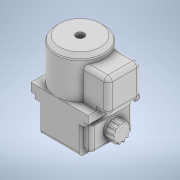
# Autodesk Inventor part: EG_Vacuumpump
Saved by Autodesk Inventor 2022 (Build 260153000, 153)
## iProperties
Created: 2023-07-06
Part Number: EG_Vacuumpump
Material: Generic
Document SubType Name: Modeling
Designer: grees
Density: 1 g/cm^3
Appearance: Default
Author: grees
Autodesk Inventor part; units mm, degrees
ref_plane "YZ Plane" through (0, 0, 0) normal (1, 0, 0) x (0, 1, 0)
ref_plane "XZ Plane" through (0, 0, 0) normal (0, 1, 0) x (-1, 0, 0)
ref_plane "XY Plane" through (0, 0, 0) normal (0, 0, 1) x (1, 0, 0)
sketch "Sketch1" plane through (0, 0, 0) normal (0, 1, 0) x (-1, 0, 0)
  circle A0 centre (0, 0) radius 30
  dimension "d0" = 60
  constraints: 1 centre point, 1 coincident
  measures "d0" diameter of A0
extrude "Extrusion1" add sketch "Sketch1" along normal blind 10
chamfer "Chamfer1" distance 5 angle 45 1 edges at (30, 10, 0)
sketch "Sketch2" plane through (0, 0, 0) normal (0, -1, 0) x (1, 0, 0)
  circle A0 centre (0, 0) radius 30
  dimension "d9" = 60
  constraints: 1 centre point, 1 coincident
  measures "d9" diameter of A0
extrude "Extrusion2" add sketch "Sketch2" along normal blind 40
chamfer "Chamfer3" distance 1 angle 45 1 edges at (30, 5, 0)
sketch "Sketch3" plane through (0, -40, 0) normal (0, -1, 0) x (1, 0, 0)
  circle A0 centre (0, 0) radius 30 projected
  line L0 (-30, 0) -> (-30, 30)
  line L1 (-30, 0) -> (-30, -30)
  line L2 (-30, -30) -> (40, -30)
  line L3 (40, -30) -> (40, 30)
  line L4 (40, 30) -> (-30, 30)
  dimension "d15" = 30
  dimension "d16" = 30
  dimension "d17" = 70
  dimension "d18" = 60
  constraints: 10 end point, 3 vertical, 2 perpendicular, 1 horizontal alignment, 1 other
  measures "d15" distance of L0.start L0.end
  measures "d16" distance of L0.start L1.end
  measures "d17" distance of L1.end L2.end
  measures "d18" distance of L2.end L3.end
extrude "Extrusion3" add sketch "Sketch3" along normal blind 10
sketch "Sketch4" plane through (0, -50, 0) normal (0, -1, 0) x (1, 0, 0)
  line L0 (40, 30) -> (-30, 30) projected
  line L1 (-30, 30) -> (-25, 30)
  line L2 (-25, 30) -> (-25, -30)
  line L3 (-30, -30) -> (40, -30) projected
  line L4 (-25, -30) -> (35, -30)
  line L5 (0, -30) -> (40, -30) projected
  line L6 (35, -30) -> (35, 30)
  line L7 (35, 30) -> (-25, 30)
  point P0 (0, 0)
  dimension "d21" = 5
  dimension "d22" = 60
  constraints: 10 end point, 4 point on line, 2 perpendicular, 1 collinear
  measures "d21" distance of L0.end L1.end
  measures "d22" distance of L2.end L4.end
extrude "Extrusion4" add sketch "Sketch4" along normal blind 5
sketch "Sketch5" plane through (0, -55, 0) normal (0, -1, 0) x (1, 0, 0)
  line L0 (-25, -30) -> (-25, 30) projected
  line L1 (-25, 30) -> (-18, 30)
  line L2 (0, 30) -> (-30, 30) projected
  line L3 (-18, 30) -> (-18, -30)
  line L4 (-25, -30) -> (35, -30) projected
  line L5 (-18, -30) -> (29, -30)
  line L6 (29, -30) -> (29, 30)
  line L7 (40, 30) -> (0, 30) projected
  line L8 (29, 30) -> (-18, 30)
  point P0 (0, 0)
  dimension "d25" = 7
  dimension "d26" = 47
  constraints: 10 end point, 4 point on line, 3 perpendicular
  measures "d25" distance of L0.end L1.end
  measures "d26" distance of L3.end L5.end
extrude "Extrusion5" add sketch "Sketch5" along normal blind 35 contours L3 L2 L7 L6 L4
fillet "Fillet1" radius 5 1 edges at (5.5, -90, 30)
fillet "Fillet2" radius 5 1 edges at (5.5, -90, -30)
sketch "Sketch6" plane through (0, -90, 0) normal (0, -1, 0) x (1, 0, 0)
  circle A0 centre (0, 0) radius 10
  dimension "d31" = 20
  constraints: 1 centre point, 1 coincident
  measures "d31" diameter of A0
extrude "Extrusion6" cut sketch "Sketch6" against normal blind 35
sketch "Sketch7" plane through (29, -55, 30) normal (1, 0, 0) x (0, 0, -1)
  line L0 (0, 0) -> (0, -35) projected
  line L1 (0, 0) -> (5, 0)
  line L2 (40, 0) -> (20, 0) projected
  line L3 (5, 0) -> (5, -30)
  line L4 (5, -30) -> (55, -30)
  line L5 (55, -30) -> (55, 0)
  line L6 (0, 0) -> (60, 0) projected
  line L7 (55, 0) -> (5, 0)
  point P0 (30, 55)
  point P1 (0, -30)
  dimension "d34" = 5
  constraints: 10 end point, 3 perpendicular, 1 collinear, 1 point on line
  measures "d34" distance of L0.start L1.end
extrude "Extrusion7" add sketch "Sketch7" along normal blind 10
fillet "Fillet3" radius 4 1 edges at (39, -70, 25)
fillet "Fillet4" radius 4 3 edges at (39, -85, -2) (37.8284, -85, 23.8284) (32, -85, 25)
fillet "Fillet5" radius 4 3 edges at (39, -68, -25) (37.8284, -83.8284, -25) (32, -85, -25)
sketch "Sketch8" plane through (39, -55, 30) normal (1, 0, 0) x (0, 0, -1)
  circle A0 centre (30, -12.943) radius 10
  point P0 (30, 55)
  dimension "d40" = 20
  constraints: 1 centre point
  measures "d40" diameter of A0
extrude "Extrusion8" cut sketch "Sketch8" against normal blind 45
sketch "Sketch9" plane through (39, -55, 30) normal (1, 0, 0) x (0, 0, -1)
  circle A0 centre (30, -13.3001) radius 7.5
  point P0 (30, 55)
  dimension "d43" = 15
  constraints: 1 centre point
  measures "d43" diameter of A0
extrude "Extrusion10" add sketch "Sketch9" against normal blind 50
sketch "Sketch10" plane through (39, -55, 30) normal (1, 0, 0) x (0, 0, -1)
  circle A0 centre (30, -12.943) radius 11
  point P0 (30, 55)
  dimension "d48" = 22
  constraints: 1 centre point
  measures "d48" diameter of A0
extrude "Extrusion11" add sketch "Sketch10" along normal blind 2
sketch "Sketch11" plane through (41, -67.943, 0) normal (1, 0, 0) x (0, 0, -1)
  circle A0 centre (0, -0.3571) radius 7.5 projected
  circle A1 centre (0, -0.3571) radius 11
  point P0 (0, 67.943)
  dimension "d51" = 22
  constraints: 1 centre point, 1 coincident
  measures "d51" diameter of A1
extrude "Extrusion12" add sketch "Sketch11" along normal blind 10 contours A0 | A1
sketch "Sketch12" plane through (51, -68.3001, 0) normal (1, 0, 0) x (0, 0, -1)
  circle A0 centre (0, 0.3571) radius 11 projected
  line L0 (0, 11.3571) -> (0, -10.6429)
  circle A1 centre (0, 11.3571) radius 2
  circle A2 centre (-5.5, 9.8834) radius 2
  circle A3 centre (-9.5263, 5.8571) radius 2
  circle A4 centre (-11, 0.3571) radius 2
  circle A5 centre (-9.5263, -5.1429) radius 2
  circle A6 centre (-5.5, -9.1692) radius 2
  circle A7 centre (0, -10.6429) radius 2
  circle A8 centre (5.5, -9.1692) radius 2
  circle A9 centre (9.5263, -5.1429) radius 2
  circle A10 centre (11, 0.3571) radius 2
  circle A11 centre (9.5263, 5.8571) radius 2
  circle A12 centre (5.5, 9.8834) radius 2
  point P0 (0, 68.3001)
  dimension "d57" = 360
  constraints: 12 centre point, 2 end point, 2 point on circle, 1 coincident, 1 vertical, 25 other
extrude "Extrusion13" cut sketch "Sketch12" against normal blind 10 contours A0 A10 | A0 A10 | A11 A0 | A0 A11 | A9 A0 | A0 A9 | A12 A0 | A0 A12 | A8 A0 | A0 A8 | A1 L0 A0 | A0 A1 | A7 A0 | A0 L0 A7 | L0 A1 A0 | A0 A7 L0 | A2 A0 | A0 A2 | A6 A0 | A0 A6 | A3 A0 | A0 A3 | A5 A0 | A0 A5 | A4 A0 | A0 A4
sketch "Sketch13" plane through (0, -90, 0) normal (0, -1, 0) x (1, 0, 0)
  circle A0 centre (0, 0) radius 11.5
  dimension "d61" = 23
  constraints: 1 centre point, 1 coincident
  measures "d61" diameter of A0
extrude "Extrusion14" add sketch "Sketch13" along normal blind 4
sketch "Sketch14" plane through (0, -94, 0) normal (0, -1, 0) x (1, 0, 0)
  circle A0 centre (0, 0) radius 10
  dimension "d64" = 20
  constraints: 1 centre point, 1 coincident
  measures "d64" diameter of A0
extrude "Extrusion15" cut sketch "Sketch14" against normal blind 5
sketch "Sketch15" plane through (40, -40, 30) normal (1, 0, 0) x (0, 0, -1)
  circle A0 centre (54.5126, -5.7503) radius 2.5
  point P0 (30, 40)
  dimension "d67" = 5
  constraints: 1 centre point
  measures "d67" diameter of A0
extrude "Extrusion16" add sketch "Sketch15" along normal blind 2
sketch "Sketch16" plane through (40, -40, 30) normal (1, 0, 0) x (0, 0, -1)
  circle A0 centre (54.5126, -5.7503) radius 2.5 projected
  circle A1 centre (54.5126, -5.7503) radius 4
  point P0 (30, 40)
  dimension "d70" = 8
  constraints: 1 centre point, 1 coincident
  measures "d70" diameter of A1
extrude "Extrusion18" add sketch "Sketch16" along normal blind 6 contours A0 | A1
fillet "Fillet6" radius 1.5 1 edges at (46, -45.7503, -20.5126)
sketch "Sketch18" plane through (0, -40, 0) normal (0, 1, 0) x (1, 0, 0)
  line L0 (24.2354, 0) -> (24.2354, 20)
  line L1 (24.2354, 0) -> (44.2354, 0) construction
  line L2 (24.2354, 0) -> (24.2354, -20)
  line L3 (40, -30) -> (0, -30) projected
  line L4 (24.2354, -20) -> (54.2354, -20)
  line L5 (54.2354, -20) -> (54.2354, 20)
  line L6 (54.2354, 20) -> (24.2354, 20)
  point P0 (0, 0)
  dimension "d84" = 20
  dimension "d85" = 90
  dimension "d86" = 20
  dimension "d87" = 30
  constraints: 12 end point, 5 perpendicular, 1 horizontal, 1 vertical
  measures "d84" distance of L0.start L0.end
  measures "d85" angle of L1 L0
  measures "d86" distance of L0.start L2.end
  measures "d87" distance of L2.end L4.end
extrude "Extrusion20" add sketch "Sketch18" along normal blind 40
fillet "Fillet9" radius 5 1 edges at (54.2354, 0, 0)
fillet "Fillet10" radius 5 3 edges at (36.7354, 0, -20) (52.7709, -1.4645, -20) (54.2354, -22.5, -20)
fillet "Fillet11" radius 5 3 edges at (54.2354, -22.5, 20) (52.7709, -1.4645, 20) (36.7354, 0, 20)
sketch "Sketch19" plane through (0, 10, 0) normal (0, 1, 0) x (1, 0, 0)
  circle A0 centre (0, 0) radius 5
  dimension "d93" = 10
  constraints: 1 centre point, 1 coincident
  measures "d93" diameter of A0
extrude "Extrusion21" cut sketch "Sketch19" against normal blind 10
fillet "Fillet12" radius 5 5 edges at (54.2354, -40, 0) (52.7709, -40, -18.5355) (44.6177, -40, -20) (52.7709, -40, 18.5355) (44.6177, -40, 20)
body "Solid1"
